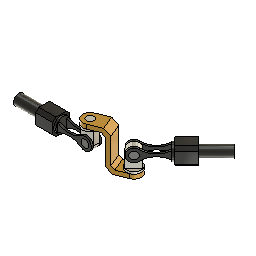
Angular Transmitter Mechanism v0 (Autodesk Fusion 360 design; units mm, degrees)
Autodesk Fusion 360 part; units mm, degrees
sketch "Sketch1" plane through (0, 0, 0) normal (0, 0, 1) x (1, 0, 0) in component "Fork"
  line L0 (20, -20) -> (-20, -20)
  line L1 (-20, -20) -> (-20, 20)
  line L2 (-20, 20) -> (20, 20)
  line L3 (20, 20) -> (20, -20)
  line L4 (20, -20) -> (-20, 20) construction
  line L5 (-20, -20) -> (20, 20) construction
  dimension "d1" = 40
  dimension "d2" = 40
  constraint horizontal L0
  constraint perpendicular L0 L1
  constraint parallel L0 L2
  constraint parallel L1 L3
  constraint coincident L4 origin
  constraint coincident L5 origin
  measures "d1" distance of L1.end L2.end
  measures "d2" distance of L0.end L1.end
extrude "Extrude1" add sketch "Sketch1" along normal mid plane 40 makes body 1 in component "Fork"
cylinder "CylinderPrimitive1" add diameter 35 height 5 placed x (0, 0, -1) y (0, 1, 0) z (1, 0, 0) at (20, 0, 0) bodies 1 in component "Fork"
cylinder "CylinderPrimitive2" add diameter 25 height 60 placed x (0, 0, 1) y (0, 1, 0) z (-1, 0, 0) at (-20, 0, 0) bodies 1 in component "Fork"
sketch "Sketch4" plane through (0, 0, 0) normal (0, 1, 0) x (1, 0, 0) in component "Fork"
  line L0 (-80, 12.5) -> (-80, -12.5)
  line L1 (25, -17.5) -> (25, 17.5)
  line L2 (20, 20) -> (-20, 20)
  line L3 (20, 20) -> (20, 17.5)
  line L4 (20, -17.5) -> (20, -20)
  line L5 (-20, -20) -> (20, -20)
  line L6 (-20, 20) -> (-20, 12.5)
  line L7 (-20, -12.5) -> (-20, -20)
  line L8 (-20, 12.5) -> (-80, 12.5)
  line L9 (-20, -12.5) -> (-80, -12.5)
  line L10 (20, -17.5) -> (25, -17.5)
  line L11 (20, 17.5) -> (25, 17.5)
  circle A0 centre (88.3842, 0) radius 15
  circle A1 centre (88.3842, 0) radius 8.75
  arc A2 (79.6752, -12.2128) -> (25, -10) centre (50.6452, -52.9223) ccw
  line L12 (25, 0) -> (52.3221, 0) construction
  arc A3 (25, 10) -> (79.6752, 12.2128) centre (50.6452, 52.9223) ccw
  dimension "d9" = 30
  dimension "d10" = 17.5
  dimension "d11" = 7.5
  dimension "d12" = 50
  constraint concentric A0 A1
  constraint coincident A0 A2.start
  constraint coincident L1 A2.end
  constraint midpoint L1 L12.start
  constraint perpendicular L1 L12
  constraint symmetric A2.end L12 A3.start
  constraint symmetric A2.start L12 A3.end
  constraint symmetric A2 L12 A3
  constraint tangent A0 A2
  constraint tangent A0 A3
  measures "d9" diameter of A0
  measures "d10" diameter of A1
  measures "d11" distance of L1.start A2.end
  measures "d12" radius of A2
extrude "Extrude2" add sketch "Sketch4" against normal blind 5 from surface at -7.5 contours L1 A0 A2 A3 | A0 bodies 1 in component "Fork"
mirror "Mirror1" about plane through (0, 0, 0) normal (0, 1, 0) of "Extrude2" in component "Fork"
extrude "Extrude3" add sketch "Sketch4" along normal mid plane 25 separate body contours A1 makes body 2 in component "Fork"
chamfer "Chamfer1" distance 7.5 angle 45 4 edges at (0, -20, 20) (0, 20, 20) (0, -20, -20) (0, 20, -20) on bodies 1 in component "Fork"
sketch "Sketch1 (2)" plane through (0, 0, 0) normal (0, 1, 0) x (1, 0, 0) in component "Rotar"
  circle A0 centre (88.3842, 0) radius 8.75
  circle A1 centre (88.3842, 0) radius 15
  line L0 (73.3842, 0) -> (103.3842, 0)
  line L1 (103.3842, 0) -> (103.3842, -30)
  line L2 (103.3842, -30) -> (73.3842, -30)
  line L3 (73.3842, -30) -> (73.3842, 0)
  dimension "d21" = 30
  dimension "d22" = 30
  dimension "d23" = 30
  constraint concentric A0 A1
  constraint horizontal L0
  constraint vertical L1
  constraint horizontal L2
  constraint vertical L3
  constraint coincident A1 L0.start
  measures "d21" diameter of A1
  measures "d22" distance of L0.start L0.end
  measures "d23" distance of L0.start L2.end
extrude "Extrude1'" add sketch "Sketch1 (2)" along normal mid plane 15 separate body contours A0 A1 L0 | A0 A1 L0 | A1 L1 L2 L3 makes body 3 in component "Rotar"
cylinder "CylinderPrimitive1'" add diameter 35 height 5 placed x (1, 0, 0) y (0, 1, 0) z (0, 0, 1) at (88.3842, 0, 30) bodies 3 in component "Rotar"
cylinder "CylinderPrimitive2'" add diameter 17.5 height 10 placed x (1, 0, 0) y (0, 1, 0) z (0, 0, 1) at (88.3842, 0, 35) bodies 3 in component "Rotar"
sketch "Sketch1 (3)" plane through (0, 0, 0) normal (0, 1, 0) x (1, 0, 0) in component "S link"
  line L0 (79.6342, -45) -> (97.1342, -45)
  line L1 (105.8842, -30) -> (103.3842, -30)
  line L2 (73.3842, -30) -> (70.8842, -30)
  line L3 (70.8842, -35) -> (79.6342, -35)
  line L4 (97.1342, -35) -> (105.8842, -35)
  circle A0 centre (88.3842, 0) radius 8.75
  arc A1 (103.3842, 0) -> (73.3842, 0) centre (88.3842, 0) ccw
  line L5 (103.3842, 0) -> (103.3842, -30)
  line L6 (73.3842, -30) -> (73.3842, 0)
  line L7 (79.6342, -35) -> (79.6342, -45)
  line L8 (97.1342, -35) -> (97.1342, -45)
  line L9 (70.8842, -30) -> (70.8842, -35)
  line L10 (105.8842, -30) -> (105.8842, -35)
  line L11 (70.8842, -35) -> (105.8842, -35)
  line L12 (105.8842, -35) -> (105.8842, -45)
  line L13 (105.8842, -45) -> (70.8842, -45)
  line L14 (70.8842, -45) -> (70.8842, -35)
  line L15 (105.8842, -35) -> (115.8842, -35)
  line L16 (115.8842, -35) -> (122.9553, -27.9289)
  line L17 (115.8842, -35) -> (105.8842, -35) construction
  line L18 (122.9553, -27.9289) -> (122.9553, 0)
  line L19 (105.8842, -45) -> (120.0263, -45)
  line L20 (120.0263, -45) -> (132.9553, -32.0711)
  line L21 (132.9553, -32.0711) -> (132.9553, 0)
  line L22 (122.9553, 0) -> (132.9553, 0)
  dimension "d30" = 35
  dimension "d31" = 10
  dimension "d32" = 10
  dimension "d33" = 135
  dimension "d34" = 10
  dimension "d35" = 10
  constraint horizontal L11
  constraint vertical L12
  constraint horizontal L13
  constraint vertical L14
  constraint coincident L3.start L9.end
  constraint coincident L4.end L10.end
  constraint perpendicular L12 L15
  constraint horizontal L17
  constraint vertical L18
  measures "d30" distance of L3.start L4.end
  measures "d31" distance of L3.start L13.end
  measures "d32" distance of L4.end L15.end
  measures "d33" angle of L16 L17
  measures "d34" distance of L15.end L16.end
  measures "d35" distance of L15
extrude "Extrude1''" add sketch "Sketch1 (3)" along normal mid plane 35 separate body contours L0 L7 L8 L11 L13 | L3 L7 L11 L13 L14 | L4 L8 L11 L12 L13 | L12 L15 L16 L18 L19 L20 L21 L22 makes body 4 in component "S link"
fillet "Fillet1" radius 17.5 2 edges at (70.8842, -17.5, 40) (70.8842, 17.5, 40) on bodies 4 in component "S link"
hole "Hole1" at (88.3842, 0, 45) direction (0, 0, -1) diameter 17.5 end through all bodies 4 in component "S link"
mirror "Mirror1'" about plane through (122.9553, 0, 0) normal (0, 0, -1) of bodies 4 makes body 5 in component "S link"
move_body "Move1" bodies 5 to x (-1, 0, 0) y (0, -1, 0) z (0, 0, 1) at (255.9105, 0, 0) in component "S link"
combine "Combine1" operation add target body 4 tool bodies 5 in component "S link"
sketch "Sketch1 (4)" plane through (-80, 0, 0) normal (-1, 0, 0) x (0, -1, 0)
  circle A0 centre (0, 0) radius 12.5
  circle A1 centre (0, 0) radius 20
  dimension "d45" = 40
  constraint coincident A0.centre A1.centre
  measures "d45" diameter of A1
extrude "Extrude1'''" add sketch "Sketch1 (4)" against normal blind 20 separate body makes body 6 in component "Component"
component "Fork" placed x (1, 0, 0) y (0, 1, 0) z (0, 0, 1) at (0, 0, 0)
component "Fork" placed x (-0.707107, -0.707107, 0) y (0.707107, -0.707107, 0) z (0, 0, 1) at (223.999, 92.7834, 0)
component "Rotar" placed x (1, 0, 0) y (0, 1, 0) z (0, 0, 1) at (0, 0, 0)
component "Rotar" placed x (0.707107, 0.707107, 0) y (0.707107, -0.707107, 0) z (0, 0, -1) at (99.0049, -32.2107, 0)
component "S link" placed x (0.92388, 0.382683, 0) y (-0.382683, 0.92388, 0) z (0, 0, 1) at (6.7278, -33.8232, 0)
component "Component" placed x (1, 0, 0) y (0, 1, 0) z (0, 0, 1) at (0, 0, 0)
component "Component" placed x (0.707107, 0.707107, 0) y (-0.707107, 0.707107, 0) z (0, 0, 1) at (322.994, 191.7784, 0)
